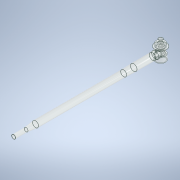
# Autodesk Inventor part: Transfer tube
Saved by Autodesk Inventor 2020 (Build 240168000, 168)
## iProperties
Created: 2020-07-11
Part Number: Transfer tube
Material: Glass
Document SubType Name: Modeling
Designer: Bruno
Density: 2.18 g/cm^3
Appearance: Clear
Author: Bruno
Autodesk Inventor part; units mm, degrees
ref_plane "YZ Plane" through (0, 0, 0) normal (1, 0, 0) x (0, 1, 0)
ref_plane "XZ Plane" through (0, 0, 0) normal (0, 1, 0) x (-1, 0, 0)
sketch "Sketch1" plane through (0, 0, 0) normal (1, 0, 0) x (0, 1, 0)
  line L0 (0, 0) -> (0, -8)
  line L1 (5.5, 0) -> (5.5, -40)
  line L2 (9, -69.9247) -> (9, -349.9247)
  line L3 (5.5, -40) -> (9, -69.9247)
  line L4 (10, -381.8231) -> (10, -441.8231)
  line L5 (10, -441.8231) -> (11, -441.8231) construction
  line L6 (10, -441.8231) -> (15, -441.8231) construction
  line L7 (9, -349.9247) -> (10, -381.8231)
  line L8 (10, -441.8231) -> (11, -450.3946)
  line L9 (11, -450.3946) -> (11, -480.3946)
  line L10 (11.95, -480.3946) -> (11.95, -450.3393)
  line L11 (11.95, -450.3393) -> (10.95, -441.7679)
  line L12 (10.95, -441.7679) -> (10.95, -381.8082)
  line L13 (10.95, -381.8082) -> (9.95, -349.9098)
  line L14 (9.95, -349.9098) -> (9.95, -69.8693)
  line L15 (9.95, -69.8693) -> (6.45, -39.9445)
  line L16 (6.45, -39.9445) -> (6.4387, -0.9497)
  line L17 (11, -480.3946) -> (11.95, -480.3946)
  line L18 (6.4387, -0.9497) -> (6.4387, 0)
  line L19 (6.4387, 0) -> (5.5, 0)
  dimension "d0" = 8
  dimension "d1" = 40
  dimension "d2" = 5.5
  dimension "d4" = 280
  dimension "d5" = 9
  dimension "d8" = 60
  dimension "d11" = 10
  dimension "d21" = 30
  dimension "d22" = 0.95
  constraints: 40 end point, 6 vertical, 3 horizontal, 1 perpendicular, 5 other
  measures "d0" distance of L0.start L0.end
  measures "d1" distance of L1.start L1.end
  measures "d2" distance between parallel lines of L0 L1
  measures "d4" distance of L2.start L2.end
  measures "d5" distance between parallel lines of L0 L2
  measures "d8" distance of L4.start L4.end
  measures "d11" distance between parallel lines of L0 L4
  measures "d21" distance of L8.end L9.end
  measures "d22" distance between parallel lines of L4 L12
revolve "Revolution1" add sketch "Sketch1" angle 360 about axis through (0, 0, 0) along (0, 0, -1)
sketch "Sketch2" plane through (0, 0, 0) normal (1, 0, 0) x (0, 1, 0)
  point P0 (0, 0)
sketch "Sketch3" plane through (0, 0, 0) normal (0, 1, 0) x (-1, 0, 0)
  circle A0 centre (0, -467.3946) radius 12
  line L0 (-11.95, -480.3946) -> (11.95, -480.3946) projected
  circle A1 centre (0, -467.3946) radius 10
  line L1 (11.95, -450.3393) -> (11.95, -480.3946) projected
  line L2 (11.95, -466.3003) -> (11.95, -480.3946)
  line L3 (-11.95, -450.3393) -> (-11.95, -480.3946) projected
  line L4 (-11.95, -466.3003) -> (-11.95, -480.3946)
  line L5 (-11.95, -480.3946) -> (11.95, -480.3946)
  point P0 (0, 0)
  point P1 (-11.95, -468.4889)
  point P2 (11.95, -468.4889)
  dimension "d23" = 24
  dimension "d24" = 13
  dimension "d25" = 20
  constraints: 6 end point, 3 collinear, 2 centre point, 2 point on circle, 2 point on line, 1 coincident
  measures "d23" diameter of A0
  measures "d24" distance from line of A0.centre L0
  measures "d25" diameter of A1
extrude "Extrusion1" cut sketch "Sketch3" against normal through all both and the other way through all contours L1 L0 L3 A0 | A1
sketch "Sketch4" plane through (0, 0, 0) normal (0, 1, 0) x (-1, 0, 0)
  circle A0 centre (0, -467.3946) radius 12
  circle A1 centre (0, -467.3946) radius 10
  point P0 (0, 0)
  point P1 (0, 0)
  point P2 (-11.95, -468.4889)
  point P3 (11.95, -468.4889)
  dimension "d28" = 24
  dimension "d30" = 20
  constraints: 2 centre point, 1 coincident
  measures "d28" diameter of A0
  measures "d30" diameter of A1
extrude "Extrusion2" add sketch "Sketch4" along normal blind 15 and the other way blind 4
sketch "Sketch5" plane through (0, -4, 0) normal (0, -1, 0) x (1, 0, 0)
  circle A0 centre (0, -467.3946) radius 10 projected
  circle A1 centre (0, -467.3946) radius 13
  circle A2 centre (0, -467.3946) radius 15.5
  point P0 (0, 0)
  dimension "d35" = 26
  dimension "d36" = 31
  constraints: 2 centre point, 2 coincident
  measures "d35" diameter of A1
  measures "d36" diameter of A2
extrude "Extrusion3" cut sketch "Sketch5" along normal through all contours A1
sketch "Sketch6" plane through (0, -4, 0) normal (0, -1, 0) x (1, 0, 0)
  circle A0 centre (0, -467.3946) radius 10
  circle A1 centre (0, -467.3946) radius 13
  circle A2 centre (0, -467.3946) radius 15.5
  point P0 (0, 0)
  point P1 (0, 0)
  dimension "d39" = 26
  dimension "d40" = 31
  constraints: 3 centre point, 2 coincident
  measures "d39" diameter of A1
  measures "d40" diameter of A2
extrude "Extrusion4" add sketch "Sketch6" along normal blind 2 contours A1 | A2
sketch "Sketch7" plane through (0, -6, 0) normal (0, -1, 0) x (1, 0, 0)
  circle A0 centre (0, -467.3946) radius 10
  circle A1 centre (0, -467.3946) radius 13
  circle A2 centre (0, -467.3946) radius 15.5
  point P0 (0, 0)
  point P1 (0, 0)
  point P2 (0, 0)
  dimension "d43" = 26
  dimension "d44" = 31
  constraints: 3 centre point, 2 coincident
  measures "d43" diameter of A1
  measures "d44" diameter of A2
extrude "Extrusion5" add sketch "Sketch7" along normal blind 15 contours A2
sketch "Sketch8" plane through (0, 15, -467.3946) normal (0, 1, 0) x (1, 0, 0)
  circle A0 centre (0, 0) radius 6
  circle A1 centre (0, 0) radius 18.5
  point P0 (0, -467.3946)
  dimension "d47" = 12
  dimension "d48" = 37
  constraints: 2 centre point, 1 coincident
  measures "d47" diameter of A0
  measures "d48" diameter of A1
extrude "Extrusion6" add sketch "Sketch8" along normal blind 2
sketch "Sketch9" plane through (0, 17, -467.3946) normal (0, 1, 0) x (1, 0, 0)
  circle A0 centre (0, 0) radius 6 projected
  circle A1 centre (0, 0) radius 6
  circle A2 centre (0, 0) radius 14
  point P0 (0, -467.3946)
  dimension "d51" = 12
  dimension "d52" = 28
  constraints: 2 centre point, 2 coincident
  measures "d51" diameter of A1
  measures "d52" diameter of A2
extrude "Extrusion7" add sketch "Sketch9" along normal blind 8
sketch "Sketch10" plane through (0, 25, -467.3946) normal (0, 1, 0) x (1, 0, 0)
  circle A0 centre (0, 0) radius 6
  circle A1 centre (0, 0) radius 7
  point P0 (0, -467.3946)
  dimension "d55" = 14
  constraints: 2 centre point, 1 coincident
  measures "d55" diameter of A1
extrude "Extrusion8" add sketch "Sketch10" along normal blind 11
sketch "Sketch11" plane through (0, -21, -467.3946) normal (0, -1, 0) x (1, 0, 0)
  line L0 (0, 0) -> (0, 15.5)
  circle A0 centre (0, 0) radius 15.5 projected
  point P0 (0, 467.3946)
  constraints: 2 end point, 1 vertical, 1 vertical alignment, 1 other
ref_plane "Work Plane1" through (0, -21, -451.8946) normal (0, 0, 1) x (1, 0, 0)
sketch "Sketch12" plane through (0, -21, -451.8946) normal (0, 0, 1) x (1, 0, 0)
  circle A0 centre (0, 21) radius 9 projected
  circle A1 centre (0, 21) radius 11
  point P0 (0, 21)
  dimension "d58" = 22
  constraints: 1 centre point, 1 coincident
  measures "d58" diameter of A1
extrude "Extrusion9" cut sketch "Sketch12" against normal blind 10 contours A0
body "Solid1"
